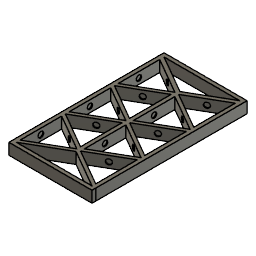
Final Assembly (Autodesk Fusion 360 archive; units mm, degrees)
design "Divider"
Autodesk Fusion 360 part; units mm, degrees
sketch "Sketch1" plane through (0, 0, 0) normal (0, 1, 0) x (1, 0, 0) in component "Divider"
  line L0 (0, 0) -> (127.3337, 73.5162)
  line L1 (0, 12.7) -> (120.9837, 82.55)
  line L2 (120.9837, 82.55) -> (0, 152.4)
  line L3 (0, 152.4) -> (0, 12.7)
  line L4 (127.3337, 73.5162) -> (127.3337, 423.7485) construction
  line L5 (120.9837, 95.25) -> (0, 165.1)
  line L6 (0, 165.1) -> (120.9837, 234.95)
  line L7 (120.9837, 234.95) -> (120.9837, 95.25)
  line L8 (120.9837, 247.65) -> (0, 177.8)
  line L9 (0, 177.8) -> (0, 317.5)
  line L10 (0, 317.5) -> (120.9837, 247.65)
  line L11 (0, 330.2) -> (120.9837, 260.35)
  line L12 (120.9837, 260.35) -> (120.9837, 400.05)
  line L13 (120.9837, 400.05) -> (0, 330.2)
  line L14 (0, 342.9) -> (120.9837, 412.75)
  line L15 (120.9837, 412.75) -> (0, 482.6)
  line L16 (0, 482.6) -> (0, 342.9)
  line L17 (127.3337, 423.7485) -> (0, 497.2647)
  line L18 (0, -12.7) -> (-12.7, -12.7)
  line L19 (-12.7, -12.7) -> (-12.7, 0)
  line L20 (-12.7, 497.2647) -> (-12.7, 509.9647)
  line L21 (0, 509.9647) -> (-12.7, 509.9647)
  line L22 (-12.7, 497.2647) -> (-12.7, 0)
  line L23 (254.6675, 12.7) -> (133.6837, 82.55)
  line L24 (254.6675, 482.6) -> (254.6675, 342.9)
  line L25 (127.3337, 423.7485) -> (254.6675, 497.2647)
  line L26 (133.6837, 412.75) -> (254.6675, 482.6)
  line L27 (133.6837, 400.05) -> (254.6675, 330.2)
  line L28 (267.3675, -12.7) -> (267.3675, 0)
  line L29 (133.6837, 247.65) -> (254.6675, 177.8)
  line L30 (254.6675, 177.8) -> (254.6675, 317.5)
  line L31 (267.3675, 497.2647) -> (267.3675, 0)
  line L32 (254.6675, 509.9647) -> (267.3675, 509.9647)
  line L33 (254.6675, 165.1) -> (133.6837, 234.95)
  line L34 (254.6675, -12.7) -> (267.3675, -12.7)
  line L35 (254.6675, 0) -> (127.3337, 73.5162)
  line L36 (254.6675, 317.5) -> (133.6837, 247.65)
  line L37 (254.6675, 330.2) -> (133.6837, 260.35)
  line L38 (133.6837, 234.95) -> (133.6837, 95.25)
  line L39 (254.6675, 152.4) -> (254.6675, 12.7)
  line L40 (267.3675, 497.2647) -> (267.3675, 509.9647)
  line L41 (133.6837, 82.55) -> (254.6675, 152.4)
  line L42 (254.6675, 342.9) -> (133.6837, 412.75)
  line L43 (133.6837, 260.35) -> (133.6837, 400.05)
  line L44 (133.6837, 95.25) -> (254.6675, 165.1)
  line L45 (0, 497.2647) -> (254.6675, 497.2647)
  line L46 (0, 0) -> (254.6675, 0)
  line L47 (0, -12.7) -> (254.6675, -12.7)
  line L48 (0, 509.9647) -> (254.6675, 509.9647)
  point P0 (254.6675, 0)
  dimension "d7" = 139.7
  dimension "d8" = 139.7
  dimension "d9" = 60
  dimension "d10" = 12.7
  dimension "d12" = 127.3337
  dimension "d14" = 139.7
  dimension "d15" = 139.7
  dimension "d16" = 12.7
  dimension "d17" = 12.7
  dimension "d19" = 139.7
  dimension "d20" = 139.7
  dimension "d21" = 139.7
  dimension "d22" = 6.35
  dimension "d23" = 12.7
  dimension "d24" = 12.7
  dimension "d26" = 139.7
  dimension "d27" = 139.7
  dimension "d28" = 6.35
  dimension "d29" = 12.7
  dimension "d30" = 6.35
  dimension "d31" = 139.7
  dimension "d32" = 139.7
  dimension "d34" = 12.7
  dimension "d35" = 12.7
  dimension "d36" = 12.7
  dimension "d38" = 12.7
  dimension "d39" = 12.7
  dimension "d41" = 12.7
  dimension "d43" = 12.7
  dimension "d44" = 12.7
  dimension "d45" = 12.7
  dimension "d46" = 12.7
  dimension "d47" = 12.7
  dimension "d48" = 254.6675
  constraint coincident L0.start L46.start
  constraint vertical L3
  constraint vertical L0.start L1.start
  constraint parallel L0 L1
  constraint vertical L4
  constraint parallel L6 L8
  constraint vertical L9
  constraint parallel L10 L11
  constraint parallel L9 L12
  constraint parallel L13 L14
  constraint vertical L16
  constraint parallel L15 L17
  constraint vertical L15.end L17.end
  constraint perpendicular L20 L21
  constraint perpendicular L18 L22
  constraint symmetric L0.start L4 L35.start
  constraint symmetric L0.start L4 P0
  constraint symmetric L0.end L4 L35.end
  constraint symmetric L1.start L4 L23.start
  constraint symmetric L1.end L4 L23.end
  constraint symmetric L2.end L4 L39.start
  constraint symmetric L4 L5.start L38.end
  constraint symmetric L4 L5.end L33.start
  constraint symmetric L4 L6.end L33.end
  constraint symmetric L4 L8.start L29.start
  constraint symmetric L4 L8.end L29.end
  constraint symmetric L4 L9.end L30.end
  constraint symmetric L4 L11.start L27.end
  constraint symmetric L4 L11.end L37.end
  constraint symmetric L4 L12.end L27.start
  constraint symmetric L4 L14.start L24.end
  constraint symmetric L4 L14.end L26.start
  constraint symmetric L4 L15.end L24.start
  constraint symmetric L4 L17.start L25.start
  constraint symmetric L4 L17.end L25.end
  constraint symmetric L4 L19.end L28.end
  constraint symmetric L4 L18.start L34.start
  constraint symmetric L4 L18.end L28.start
  constraint symmetric L4 L21.start L32.start
  constraint symmetric L4 L20.start L31.start
  constraint symmetric L4 L20.end L32.end
  constraint coincident P0 L35.start
  constraint parallel L32 L48
  measures "d7" distance of L1.start L1.end
  measures "d8" distance of L1.end L2.end
  measures "d9" angle of L2 L3
  measures "d10" vertical distance of L0.start L1.start
  measures "d12" horizontal distance of L0.start L0.end
  measures "d14" distance of L5.end L6.end
  measures "d15" vertical distance of L5.start L6.end
  measures "d16" vertical distance of L1.end L5.start
  measures "d17" distance of L2.end L5.end
  measures "d19" distance of L5.start L5.end
  measures "d20" distance of L8.start L8.end
  measures "d21" distance of L8.end L9.end
  measures "d22" distance of L4 L8.start
  measures "d23" distance of L5.end L8.end
  measures "d24" distance of L9.end L11.start
  measures "d26" distance of L11.start L12.end
  measures "d27" distance of L11.start L11.end
  measures "d28" distance of L4 L12.end
  measures "d29" distance of L11.start L14.start
  measures "d30" distance of L4 L14.end
  measures "d31" distance of L14.start L15.end
  measures "d32" distance of L14.end L15.end
  measures "d34" distance of L15 L17
  measures "d35" distance of L0.start L19.end
  measures "d36" distance of L0.start L18.start
  measures "d38" distance of L17.end L21.start
  measures "d39" distance of L17.end L20.start
  measures "d41" distance of L31 L39
  measures "d43" distance of L32.end L31.start
  measures "d44" distance of L32.end L32.start
  measures "d45" distance of L19.end L18.end
  measures "d46" distance of L18.start L18.end
  measures "d47" distance of L7 L38
  measures "d48" distance of L18.start L34.start
extrude "Extrude1" add sketch "Sketch1" along normal blind 38.1 in component "Divider"
sketch "Sketch2" plane through (0, 0, 0) normal (1, 0, 0) x (0, 0, -1) in component "Divider"
  line L0 (177.8, 0) -> (317.5, 0)
  line L1 (317.5, 0) -> (317.5, 38.1)
  line L2 (317.5, 38.1) -> (177.8, 38.1)
  line L3 (177.8, 38.1) -> (177.8, 0)
  line L4 (12.7, 38.1) -> (152.4, 38.1)
  line L5 (177.8, 38.1) -> (317.5, 38.1)
  line L6 (342.9, 38.1) -> (482.6, 38.1)
  line L7 (177.8, 0) -> (317.5, 0)
  line L8 (342.9, 0) -> (482.6, 0)
  line L9 (12.7, 0) -> (152.4, 0)
  circle A0 centre (412.75, 19.05) radius 8.89
  circle A1 centre (247.65, 19.05) radius 8.89
  circle A2 centre (82.55, 19.05) radius 9.525
  dimension "d61" = 17.78
  dimension "d62" = 69.85
  dimension "d63" = 19.05
  dimension "d64" = 17.78
  dimension "d65" = 19.05
  dimension "d66" = 69.85
  dimension "d67" = 19.05
  dimension "d68" = 19.05
  dimension "d69" = 69.85
  measures "d61" diameter of A0
  measures "d62" horizontal distance of L6.end A0.centre
  measures "d63" distance of L6 A0.centre
  measures "d64" diameter of A1
  measures "d65" distance of L2 A1.centre
  measures "d66" horizontal distance of L2.end A1.centre
  measures "d67" diameter of A2
  measures "d68" vertical distance of L4.end A2.centre
  measures "d69" horizontal distance of L4.start A2.centre
extrude "Extrude2" cut sketch "Sketch2" against normal blind 3.048 contours A0 | A1 | A2 in component "Divider"
sketch "Sketch2 (1)" plane through (254.6675, 0, 0) normal (-1, 0, 0) x (0, 0, 1) in component "Divider"
  line L0 (-317.5, 0) -> (-177.8, 0)
  line L1 (-177.8, 0) -> (-177.8, 38.1)
  line L2 (-177.8, 38.1) -> (-317.5, 38.1)
  line L3 (-317.5, 38.1) -> (-317.5, 0)
  line L4 (-482.6, 38.1) -> (-342.9, 38.1)
  line L5 (-482.6, 0) -> (-342.9, 0)
  line L6 (-317.5, 0) -> (-177.8, 0)
  line L7 (-317.5, 38.1) -> (-177.8, 38.1)
  line L8 (-152.4, 38.1) -> (-12.7, 38.1)
  line L9 (-152.4, 0) -> (-12.7, 0)
  circle A0 centre (-82.55, 19.05) radius 8.89
  circle A1 centre (-247.65, 19.05) radius 8.89
  circle A2 centre (-412.75, 19.05) radius 8.89
  dimension "d72" = 17.78
  dimension "d73" = 19.05
  dimension "d74" = 69.85
  dimension "d75" = 17.78
  dimension "d76" = 19.05
  dimension "d77" = 69.85
  dimension "d78" = 17.78
  dimension "d79" = 19.05
  dimension "d80" = 69.85
  measures "d72" diameter of A0
  measures "d73" vertical distance of L8.end A0.centre
  measures "d74" horizontal distance of L8.end A0.centre
  measures "d75" diameter of A1
  measures "d76" vertical distance of L1.end A1.centre
  measures "d77" horizontal distance of L1.end A1.centre
  measures "d78" diameter of A2
  measures "d79" vertical distance of L4.end A2.centre
  measures "d80" horizontal distance of L4.end A2.centre
extrude "Extrude3" cut sketch "Sketch2 (1)" against normal blind 3.048 contours A0 | A1 | A2 in component "Divider"
sketch "Sketch3" plane through (133.6837, 0, 0) normal (1, 0, 0) x (0, 0, -1) in component "Divider"
  line L0 (95.25, 0) -> (234.95, 0)
  line L1 (234.95, 0) -> (234.95, 38.1)
  line L2 (234.95, 38.1) -> (95.25, 38.1)
  line L3 (95.25, 38.1) -> (95.25, 0)
  line L4 (95.25, 38.1) -> (234.95, 38.1)
  line L5 (95.25, 0) -> (234.95, 0)
  line L6 (260.35, 38.1) -> (400.05, 38.1)
  line L7 (260.35, 0) -> (400.05, 0)
  circle A0 centre (165.1, 19.05) radius 8.89
  circle A1 centre (330.2, 19.05) radius 8.89
  dimension "d83" = 17.78
  dimension "d84" = 19.05
  dimension "d85" = 69.85
  dimension "d86" = 17.78
  dimension "d87" = 19.05
  dimension "d88" = 69.85
  measures "d83" diameter of A0
  measures "d84" vertical distance of L1.end A0.centre
  measures "d85" horizontal distance of L2.end A0.centre
  measures "d86" diameter of A1
  measures "d87" vertical distance of L6.start A1.centre
  measures "d88" horizontal distance of L6.end A1.centre
extrude "Extrude4" cut sketch "Sketch3" against normal blind 3.048 contours A0 | A1 in component "Divider"
sketch "Sketch4" plane through (120.9837, 0, 0) normal (-1, 0, 0) x (0, 0, 1) in component "Divider"
  line L0 (-400.05, 0) -> (-260.35, 0)
  line L1 (-260.35, 0) -> (-260.35, 38.1)
  line L2 (-260.35, 38.1) -> (-400.05, 38.1)
  line L3 (-400.05, 38.1) -> (-400.05, 0)
  circle A0 centre (-330.2, 19.05) radius 8.89
  line L4 (-400.05, 38.1) -> (-260.35, 38.1)
  line L5 (-400.05, 0) -> (-260.35, 0)
  line L6 (-234.95, 0) -> (-95.25, 0)
  line L7 (-234.95, 38.1) -> (-95.25, 38.1)
  circle A1 centre (-165.1, 19.05) radius 8.89
  dimension "d91" = 17.78
  dimension "d92" = 19.05
  dimension "d93" = 69.85
  dimension "d94" = 17.78
  dimension "d95" = 19.05
  dimension "d96" = 69.85
  measures "d91" diameter of A0
  measures "d92" vertical distance of L2.end A0.centre
  measures "d93" horizontal distance of L2.end A0.centre
  measures "d94" diameter of A1
  measures "d95" vertical distance of L7.end A1.centre
  measures "d96" horizontal distance of L7.end A1.centre
extrude "Extrude5" cut sketch "Sketch4" against normal blind 3.048 contours A0 | A1 in component "Divider"
sketch "Sketch7" plane through (-71.4904, 0, -123.825) normal (0.5, 0, 0.866025) x (0.866025, 0, -0.5) in component "Divider"
  line L0 (82.55, 0) -> (222.25, 0)
  line L1 (222.25, 0) -> (222.25, 38.1)
  line L2 (222.25, 38.1) -> (82.55, 38.1)
  line L3 (82.55, 38.1) -> (82.55, 0)
  line L4 (82.55, 38.1) -> (222.25, 38.1)
  line L5 (82.55, 0) -> (222.25, 0)
  circle A0 centre (158.75, 19.05) radius 8.89
  dimension "d99" = 17.78
  dimension "d100" = 63.5
  dimension "d101" = 19.05
  measures "d99" diameter of A0
  measures "d100" horizontal distance of L1.end A0.centre
  measures "d101" vertical distance of L2.end A0.centre
extrude "Extrude6" cut sketch "Sketch7" against normal blind 3.048 contours A0 in component "Divider"
sketch "Sketch8" plane through (-142.9808, 0, -247.65) normal (0.5, 0, 0.866025) x (0.866025, 0, -0.5) in component "Divider"
  line L0 (165.1, 0) -> (304.8, 0)
  line L1 (304.8, 0) -> (304.8, 38.1)
  line L2 (304.8, 38.1) -> (165.1, 38.1)
  line L3 (165.1, 38.1) -> (165.1, 0)
  line L4 (165.1, 38.1) -> (304.8, 38.1)
  line L5 (165.1, 0) -> (304.8, 0)
  circle A0 centre (234.95, 19.05) radius 8.89
  dimension "d104" = 17.78
  dimension "d105" = 19.05
  dimension "d106" = 69.85
  measures "d104" diameter of A0
  measures "d105" vertical distance of L2.end A0.centre
  measures "d106" horizontal distance of L2.end A0.centre
extrude "Extrude7" cut sketch "Sketch8" against normal blind 3.048 contours A0 in component "Divider"
sketch "Sketch9" plane through (-2.3243, 0, -4.0257) normal (0.5, 0, 0.866025) x (0.866025, 0, -0.5) in component "Divider"
  line L0 (157.0485, 0) -> (296.7485, 0)
  line L1 (296.7485, 0) -> (296.7485, 38.1)
  line L2 (296.7485, 38.1) -> (157.0485, 38.1)
  line L3 (157.0485, 38.1) -> (157.0485, 0)
  line L4 (157.0485, 38.1) -> (296.7485, 38.1)
  line L5 (157.0485, 0) -> (296.7485, 0)
  circle A0 centre (226.8985, 19.05) radius 8.89
  dimension "d109" = 17.78
  dimension "d110" = 19.05
  dimension "d111" = 69.85
  measures "d109" diameter of A0
  measures "d110" vertical distance of L1.end A0.centre
  measures "d111" horizontal distance of L1.end A0.centre
extrude "Extrude8" cut sketch "Sketch9" against normal blind 3.048 contours A0 in component "Divider"
sketch "Sketch10" plane through (-73.8147, 0, -127.8507) normal (0.5, 0, 0.866025) x (0.866025, 0, -0.5) in component "Divider"
  line L0 (239.5985, 0) -> (379.2985, 0)
  line L1 (379.2985, 0) -> (379.2985, 38.1)
  line L2 (379.2985, 38.1) -> (239.5985, 38.1)
  line L3 (239.5985, 38.1) -> (239.5985, 0)
  line L4 (239.5985, 38.1) -> (379.2985, 38.1)
  line L5 (239.5985, 0) -> (379.2985, 0)
  circle A0 centre (309.4485, 19.05) radius 8.89
  dimension "d114" = 17.78
  dimension "d115" = 19.05
  dimension "d116" = 69.85
  measures "d114" diameter of A0
  measures "d115" vertical distance of L1.end A0.centre
  measures "d116" horizontal distance of L1.end A0.centre
extrude "Extrude9" cut sketch "Sketch10" against normal blind 3.048 contours A0 in component "Divider"
sketch "Sketch11" plane through (-145.3051, 0, -251.6757) normal (0.5, 0, 0.866025) x (0.866025, 0, -0.5) in component "Divider"
  line L0 (322.1485, 0) -> (461.8485, 0)
  line L1 (461.8485, 0) -> (461.8485, 38.1)
  line L2 (461.8485, 38.1) -> (322.1485, 38.1)
  line L3 (322.1485, 38.1) -> (322.1485, 0)
  line L4 (322.1485, 38.1) -> (461.8485, 38.1)
  line L5 (322.1485, 0) -> (461.8485, 0)
  circle A0 centre (391.9985, 19.05) radius 8.89
  dimension "d119" = 17.78
  dimension "d120" = 19.05
  dimension "d121" = 69.85
  measures "d119" diameter of A0
  measures "d120" vertical distance of L1.end A0.centre
  measures "d121" horizontal distance of L1.end A0.centre
extrude "Extrude10" cut sketch "Sketch11" against normal blind 3.048 contours A0 in component "Divider"
sketch "Sketch3 (2)" plane through (212.1469, 0, -367.4493) normal (0.5, 0, -0.866025) x (-0.866025, 0, -0.5) in component "Divider"
  line L0 (-49.0985, 0) -> (90.6015, 0)
  line L1 (90.6015, 0) -> (90.6015, 38.1)
  line L2 (90.6015, 38.1) -> (-49.0985, 38.1)
  line L3 (-49.0985, 38.1) -> (-49.0985, 0)
  line L4 (-49.0985, 38.1) -> (90.6015, 38.1)
  line L5 (-49.0985, 0) -> (90.6015, 0)
  circle A0 centre (20.7515, 19.05) radius 8.89
  dimension "d124" = 17.78
  dimension "d125" = 19.05
  dimension "d126" = 69.85
  measures "d124" diameter of A0
  measures "d125" distance of L4 A0.centre
  measures "d126" horizontal distance of L1.end A0.centre
extrude "Extrude11" cut sketch "Sketch3 (2)" against normal blind 3.048 contours A0 in component "Divider"
sketch "Sketch4 (2)" plane through (140.6565, 0, -243.6243) normal (0.5, 0, -0.866025) x (-0.866025, 0, -0.5) in component "Divider"
  line L0 (-131.6485, 0) -> (8.0515, 0)
  line L1 (8.0515, 0) -> (8.0515, 38.1)
  line L2 (8.0515, 38.1) -> (-131.6485, 38.1)
  line L3 (-131.6485, 38.1) -> (-131.6485, 0)
  line L4 (-131.6485, 38.1) -> (8.0515, 38.1)
  line L5 (-131.6485, 0) -> (8.0515, 0)
  circle A0 centre (-61.7985, 19.05) radius 8.89
  dimension "d129" = 17.78
  dimension "d130" = 19.05
  dimension "d131" = 69.85
  measures "d129" diameter of A0
  measures "d130" distance of L2 A0.centre
  measures "d131" horizontal distance of L1.end A0.centre
extrude "Extrude12" cut sketch "Sketch4 (2)" against normal blind 3.048 contours A0 in component "Divider"
sketch "Sketch5" plane through (69.1661, 0, -119.7993) normal (0.5, 0, -0.866025) x (-0.866025, 0, -0.5) in component "Divider"
  line L0 (-214.1985, 0) -> (-74.4985, 0)
  line L1 (-74.4985, 0) -> (-74.4985, 38.1)
  line L2 (-74.4985, 38.1) -> (-214.1985, 38.1)
  line L3 (-214.1985, 38.1) -> (-214.1985, 0)
  line L4 (-214.1985, 38.1) -> (-74.4985, 38.1)
  line L5 (-214.1985, 0) -> (-74.4985, 0)
  circle A0 centre (-144.3485, 19.05) radius 8.89
  dimension "d134" = 17.78
  dimension "d135" = 19.05
  dimension "d136" = 69.85
  measures "d134" diameter of A0
  measures "d135" distance of L4 A0.centre
  measures "d136" horizontal distance of L1.end A0.centre
extrude "Extrude13" cut sketch "Sketch5" against normal blind 3.048 contours A0 in component "Divider"
sketch "Sketch6" plane through (142.9808, 0, -247.65) normal (0.5, 0, -0.866025) x (-0.866025, 0, -0.5) in component "Divider"
  line L0 (25.4, 0) -> (165.1, 0)
  line L1 (165.1, 0) -> (165.1, 38.1)
  line L2 (165.1, 38.1) -> (25.4, 38.1)
  line L3 (25.4, 38.1) -> (25.4, 0)
  line L4 (25.4, 38.1) -> (165.1, 38.1)
  line L5 (25.4, 0) -> (165.1, 0)
  circle A0 centre (95.25, 19.05) radius 8.89
  dimension "d139" = 17.78
  dimension "d140" = 19.05
  dimension "d141" = 69.85
  measures "d139" diameter of A0
  measures "d140" distance of L2 A0.centre
  measures "d141" horizontal distance of L1.end A0.centre
extrude "Extrude14" cut sketch "Sketch6" against normal blind 3.048 contours A0 in component "Divider"
sketch "Sketch7 (2)" plane through (71.4904, 0, -123.825) normal (0.5, 0, -0.866025) x (-0.866025, 0, -0.5) in component "Divider"
  line L0 (-57.15, 0) -> (82.55, 0)
  line L1 (82.55, 0) -> (82.55, 38.1)
  line L2 (82.55, 38.1) -> (-57.15, 38.1)
  line L3 (-57.15, 38.1) -> (-57.15, 0)
  line L4 (-57.15, 38.1) -> (82.55, 38.1)
  line L5 (-57.15, 0) -> (82.55, 0)
  circle A0 centre (12.7, 19.05) radius 8.89
  dimension "d144" = 17.78
  dimension "d145" = 19.05
  dimension "d146" = 69.85
  measures "d144" diameter of A0
  measures "d145" distance of L2 A0.centre
  measures "d146" horizontal distance of L1.end A0.centre
extrude "Extrude15" cut sketch "Sketch7 (2)" against normal blind 3.048 contours A0 in component "Divider"
sketch "Sketch8 (2)" plane through (-148.4801, 0, -257.175) normal (-0.5, 0, -0.866025) x (-0.866025, 0, 0.5) in component "Divider"
  line L0 (-311.15, 0) -> (-171.45, 0)
  line L1 (-171.45, 0) -> (-171.45, 38.1)
  line L2 (-171.45, 38.1) -> (-311.15, 38.1)
  line L3 (-311.15, 38.1) -> (-311.15, 0)
  line L4 (-243.9838, 38.1) -> (10.9985, 38.1)
  line L5 (-311.15, 38.1) -> (-171.45, 38.1)
  line L6 (-311.15, 0) -> (-171.45, 0)
  circle A0 centre (-241.3, 19.05) radius 8.89
  dimension "d149" = 17.78
  dimension "d150" = 69.85
  dimension "d151" = 19.05
  measures "d149" diameter of A0
  measures "d150" horizontal distance of L1.end A0.centre
  measures "d151" distance of L5 A0.centre
extrude "Extrude16" cut sketch "Sketch8 (2)" against normal blind 3.048 contours A0 in component "Divider"
sketch "Sketch9 (2)" plane through (-76.9897, 0, -133.35) normal (-0.5, 0, -0.866025) x (-0.866025, 0, 0.5) in component "Divider"
  line L0 (-228.6, 0) -> (-88.9, 0)
  line L1 (-88.9, 0) -> (-88.9, 38.1)
  line L2 (-88.9, 38.1) -> (-228.6, 38.1)
  line L3 (-228.6, 38.1) -> (-228.6, 0)
  line L4 (-228.6, 38.1) -> (-88.9, 38.1)
  line L5 (-228.6, 0) -> (-88.9, 0)
  circle A0 centre (-158.75, 19.05) radius 8.89
  dimension "d154" = 17.78
  dimension "d155" = 19.05
  dimension "d156" = 69.85
  measures "d154" diameter of A0
  measures "d155" distance of L4 A0.centre
  measures "d156" horizontal distance of L1.end A0.centre
extrude "Extrude17" cut sketch "Sketch9 (2)" against normal blind 3.048 contours A0 in component "Divider"
sketch "Sketch10 (2)" plane through (-5.4993, 0, -9.525) normal (-0.5, 0, -0.866025) x (-0.866025, 0, 0.5) in component "Divider"
  line L0 (-146.05, 0) -> (-6.35, 0)
  line L1 (-6.35, 0) -> (-6.35, 38.1)
  line L2 (-6.35, 38.1) -> (-146.05, 38.1)
  line L3 (-146.05, 38.1) -> (-146.05, 0)
  line L4 (-146.05, 38.1) -> (-6.35, 38.1)
  line L5 (-146.05, 0) -> (-6.35, 0)
  circle A0 centre (-76.2, 19.05) radius 8.89
  dimension "d159" = 17.78
  dimension "d160" = 69.85
  dimension "d161" = 19.05
  measures "d159" diameter of A0
  measures "d160" horizontal distance of L1.end A0.centre
  measures "d161" distance of L4 A0.centre
extrude "Extrude18" cut sketch "Sketch10 (2)" against normal blind 3.048 contours A0 in component "Divider"
sketch "Sketch12" plane through (-79.3139, 0, -137.3757) normal (-0.5, 0, -0.866025) x (-0.866025, 0, 0.5) in component "Divider"
  line L0 (-385.6485, 0) -> (-245.9485, 0)
  line L1 (-245.9485, 0) -> (-245.9485, 38.1)
  line L2 (-245.9485, 38.1) -> (-385.6485, 38.1)
  line L3 (-385.6485, 38.1) -> (-385.6485, 0)
  line L4 (-385.6485, 38.1) -> (-245.9485, 38.1)
  line L5 (-385.6485, 0) -> (-245.9485, 0)
  circle A0 centre (-315.7985, 19.05) radius 8.89
  dimension "d164" = 17.78
  dimension "d165" = 19.05
  dimension "d166" = 69.85
  measures "d164" diameter of A0
  measures "d165" distance of L4 A0.centre
  measures "d166" horizontal distance of L1.end A0.centre
extrude "Extrude19" cut sketch "Sketch12" against normal blind 3.048 contours A0 in component "Divider"
sketch "Sketch13" plane through (-7.8235, 0, -13.5507) normal (-0.5, 0, -0.866025) x (-0.866025, 0, 0.5) in component "Divider"
  line L0 (-303.0985, 0) -> (-163.3985, 0)
  line L1 (-163.3985, 0) -> (-163.3985, 38.1)
  line L2 (-163.3985, 38.1) -> (-303.0985, 38.1)
  line L3 (-303.0985, 38.1) -> (-303.0985, 0)
  line L4 (-303.0985, 38.1) -> (-163.3985, 38.1)
  line L5 (-303.0985, 0) -> (-163.3985, 0)
  circle A0 centre (-233.2485, 19.05) radius 8.89
  dimension "d169" = 17.78
  dimension "d170" = 19.05
  dimension "d171" = 69.85
  measures "d169" diameter of A0
  measures "d170" distance of L4 A0.centre
  measures "d171" horizontal distance of L1.end A0.centre
extrude "Extrude20" cut sketch "Sketch13" against normal blind 3.048 contours A0 in component "Divider"
sketch "Sketch14" plane through (65.9911, 0, -114.3) normal (-0.5, 0, 0.866025) x (0.866025, 0, 0.5) in component "Divider"
  line L0 (-76.2, 0) -> (63.5, 0)
  line L1 (63.5, 0) -> (63.5, 38.1)
  line L2 (63.5, 38.1) -> (-76.2, 38.1)
  line L3 (-76.2, 38.1) -> (-76.2, 0)
  line L4 (-76.2, 38.1) -> (63.5, 38.1)
  line L5 (-76.2, 0) -> (63.5, 0)
  circle A0 centre (-6.35, 19.05) radius 8.89
  dimension "d174" = 17.78
  dimension "d175" = 69.85
  dimension "d176" = 19.05
  measures "d174" diameter of A0
  measures "d175" horizontal distance of L2.end A0.centre
  measures "d176" vertical distance of L2.end A0.centre
extrude "Extrude21" cut sketch "Sketch14" against normal blind 3.048 contours A0 in component "Divider"
sketch "Sketch15" plane through (137.4815, 0, -238.125) normal (-0.5, 0, 0.866025) x (0.866025, 0, 0.5) in component "Divider"
  line L0 (-158.75, 0) -> (-19.05, 0)
  line L1 (-19.05, 0) -> (-19.05, 38.1)
  line L2 (-19.05, 38.1) -> (-158.75, 38.1)
  line L3 (-158.75, 38.1) -> (-158.75, 0)
  line L4 (-158.75, 38.1) -> (-19.05, 38.1)
  line L5 (-158.75, 0) -> (-19.05, 0)
  circle A0 centre (-88.9, 19.05) radius 8.89
  dimension "d179" = 17.78
  dimension "d180" = 19.05
  dimension "d181" = 69.85
  measures "d179" diameter of A0
  measures "d180" vertical distance of L1.end A0.centre
  measures "d181" horizontal distance of L1.end A0.centre
extrude "Extrude22" cut sketch "Sketch15" against normal blind 3.048 contours A0 in component "Divider"
sketch "Sketch16" plane through (208.9719, 0, -361.95) normal (-0.5, 0, 0.866025) x (0.866025, 0, 0.5) in component "Divider"
  line L0 (-241.3, 0) -> (-101.6, 0)
  line L1 (-101.6, 0) -> (-101.6, 38.1)
  line L2 (-101.6, 38.1) -> (-241.3, 38.1)
  line L3 (-241.3, 38.1) -> (-241.3, 0)
  line L4 (-241.3, 38.1) -> (-101.6, 38.1)
  line L5 (-241.3, 0) -> (-101.6, 0)
  circle A0 centre (-171.45, 19.05) radius 8.89
  dimension "d184" = 17.78
  dimension "d185" = 69.85
  dimension "d186" = 19.05
  measures "d184" diameter of A0
  measures "d185" horizontal distance of L1.end A0.centre
  measures "d186" vertical distance of L1.end A0.centre
extrude "Extrude23" cut sketch "Sketch16" against normal blind 3.048 contours A0 in component "Divider"
sketch "Sketch17" plane through (206.6477, 0, -357.9243) normal (-0.5, 0, 0.866025) x (0.866025, 0, 0.5) in component "Divider"
  line L0 (-84.2515, 0) -> (55.4485, 0)
  line L1 (55.4485, 0) -> (55.4485, 38.1)
  line L2 (55.4485, 38.1) -> (-84.2515, 38.1)
  line L3 (-84.2515, 38.1) -> (-84.2515, 0)
  line L4 (-84.2515, 38.1) -> (55.4485, 38.1)
  line L5 (-84.2515, 0) -> (55.4485, 0)
  circle A0 centre (-14.4015, 19.05) radius 8.89
  dimension "d189" = 17.78
  dimension "d190" = 69.85
  dimension "d191" = 19.05
  measures "d189" diameter of A0
  measures "d190" horizontal distance of L1.end A0.centre
  measures "d191" vertical distance of L1.end A0.centre
extrude "Extrude24" cut sketch "Sketch17" against normal blind 3.048 contours A0 in component "Divider"
sketch "Sketch18" plane through (135.1573, 0, -234.0993) normal (-0.5, 0, 0.866025) x (0.866025, 0, 0.5) in component "Divider"
  line L0 (-1.7015, 0) -> (137.9985, 0)
  line L1 (137.9985, 0) -> (137.9985, 38.1)
  line L2 (137.9985, 38.1) -> (-1.7015, 38.1)
  line L3 (-1.7015, 38.1) -> (-1.7015, 0)
  line L4 (-1.7015, 38.1) -> (137.9985, 38.1)
  line L5 (-1.7015, 0) -> (137.9985, 0)
  circle A0 centre (68.1485, 19.05) radius 8.89
  dimension "d194" = 17.78
  dimension "d195" = 69.85
  dimension "d196" = 19.05
  measures "d194" diameter of A0
  measures "d195" horizontal distance of L1.end A0.centre
  measures "d196" vertical distance of L1.end A0.centre
extrude "Extrude25" cut sketch "Sketch18" against normal blind 3.048 contours A0 in component "Divider"
component "Divider" placed x (1, 0, 0) y (0, 1, 0) z (0, 0, 1) at (0, 0, 0)
equation "d12 = 4.7631397208 in + 0.25 in"
